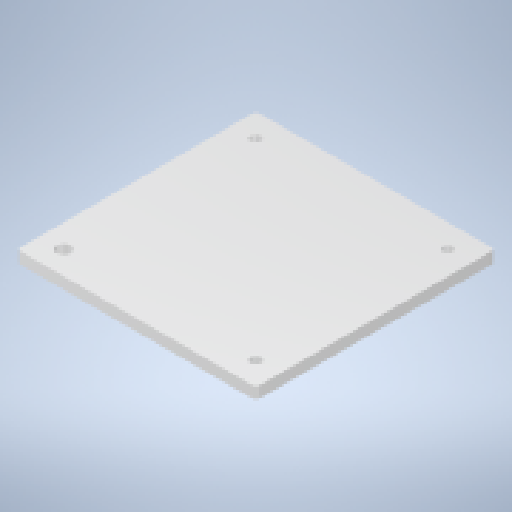
# Autodesk Inventor part: C beam gantry (small side y axis)
Saved by Autodesk Inventor 2023.2 (Build 272271000, 271)
## iProperties
Created: 2023-03-20
Part Number: C beam gantry (small side y axis)
Material: Aluminum 6061
Document SubType Name: Modeling
Designer: dmargari
Density: 2.7 g/cm^3
Appearance: Aluminum - Flat
Author: dmargari
Autodesk Inventor part; units mm, degrees
ref_plane "YZ Plane" through (0, 0, 0) normal (1, 0, 0) x (0, 1, 0)
ref_plane "XZ Plane" through (0, 0, 0) normal (0, 1, 0) x (-1, 0, 0)
ref_plane "XY Plane" through (0, 0, 0) normal (0, 0, 1) x (1, 0, 0)
sketch "Sketch1" plane through (0, 0, 0) normal (0, 1, 0) x (-1, 0, 0)
  line L0 (163.2343, -143.3167) -> (38.0343, -143.3167)
  line L1 (38.0343, -143.3167) -> (38.0343, -268.5167)
  line L2 (38.0343, -268.5167) -> (163.2343, -268.5167)
  line L3 (163.2343, -268.5167) -> (163.2343, -143.3167)
  line L4 (150.9343, -143.3167) -> (150.9343, -268.5167) construction
  line L5 (50.3343, -143.3167) -> (50.3343, -268.5167) construction
  line L6 (172.4431, -155.6167) -> (11.5351, -155.6167) construction
  line L7 (172.4431, -256.2167) -> (14.5022, -256.2167) construction
  point P0 (0, 0)
  point P1 (150.9343, -155.6167)
  point P2 (150.9343, -256.2167)
  point P3 (50.3343, -155.6167)
  point P4 (50.3343, -256.2167)
  dimension "d0" = 125.2
  dimension "d1" = 125.2
  dimension "d16" = 12.3
  dimension "d17" = 100.6
  dimension "d18" = 100.6
  constraints: 16 end point, 12 point on line, 3 horizontal, 3 perpendicular, 2 parallel
  measures "d0" distance of L2.end L1.end
  measures "d1" distance of L1.end L0.end
  measures "d16" distance between parallel lines of L0 L6
  measures "d17" distance between parallel lines of L6 L7
  measures "d18" distance between parallel lines of L5 L4
extrude "Extrusion1" add sketch "Sketch1" along normal blind 6
fillet "Fillet1" radius 2 4 edges at (-163.2343, 3, -268.5167) (-163.2343, 3, -143.3167) (-38.0343, 3, -143.3167) (-38.0343, 3, -268.5167)
hole "Hole1" at (-150.9343, 0, -256.2167) at (-50.3343, 0, -256.2167) at (-50.3343, 0, -155.6167) direction (0, 1, 0) diameter 5.1 end through all
hole "Hole2" at (-150.9343, 0, -155.6167) direction (0, 1, 0) diameter 7.2 end through all
body "Solid1"
